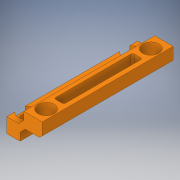
# Autodesk Inventor part: Block_3-8
Saved by Autodesk Inventor 2019 (Build 230136000, 136)
## iProperties
Created: 2019-03-07
Part Number: Block_3-8
Material: Aluminum 6061
Document SubType Name: Modeling
Designer: Delta
Density: 2.7 g/cm^3
Appearance: Orange
Mass: 102.344 g
Surface Area: 217.101 cm^2
Volume: 37.9051 cm^3
Author: Delta
Autodesk Inventor part; units mm, degrees
ref_plane "YZ Plane" through (0, 0, 0) normal (1, 0, 0) x (0, 1, 0)
ref_plane "XZ Plane" through (0, 0, 0) normal (0, 1, 0) x (-1, 0, 0)
ref_plane "XY Plane" through (0, 0, 0) normal (0, 0, 1) x (1, 0, 0)
sketch "Sketch1" plane through (0, 0, 0) normal (0, 0, 1) x (1, 0, 0)
  line L0 (0, 0) -> (0, 14.351)
  line L1 (0, 0) -> (14.351, 0) construction
  line L2 (0, 14.351) -> (16.51, 14.351)
  line L3 (16.51, 14.351) -> (16.51, 27.051)
  line L4 (16.51, 27.051) -> (34.29, 27.051)
  line L5 (34.29, 27.051) -> (34.29, 12.7)
  line L6 (34.29, 12.7) -> (12.7, 12.7)
  line L7 (12.7, 12.7) -> (12.7, 0)
  line L8 (0, 0) -> (12.7, 0)
  dimension "d0" = 14.351
  dimension "d2" = 16.51
  dimension "d6" = 17.78
  dimension "d9" = 21.59
  dimension "d47" = 14.351
  dimension "d49" = 12.7
  constraints: 18 end point, 6 perpendicular, 2 horizontal, 1 collinear, 1 point on line, 1 vertical
  measures "d0" distance of L0.start L0.end
  measures "d2" distance of L0.end L2.end
  measures "d6" distance of L3.end L4.end
  measures "d9" distance of L5.end L6.end
  measures "d47" distance of L4.end L5.end
  measures "d49" distance of L2.end L3.end
extrude "Extrusion1" add sketch "Sketch1" along normal blind 127
sketch "Sketch3" plane through (16.51, 27.051, 0) normal (0, 1, 0) x (1, 0, 0)
  line L0 (0, -127) -> (-16.51, -127) projected
  line L1 (-16.51, 0) -> (0, 0) projected
  line L2 (-16.51, 0) -> (-16.51, -127) projected
  point P0 (-10.16, -12.7)
  point P1 (-10.16, -114.3)
  dimension "d25" = 12.7
  dimension "d26" = 12.7
  dimension "d27" = 6.35
  dimension "d28" = 6.35
  measures "d25" distance from line of L0 point (-10.16, -114.3)
  measures "d26" distance from line of L1 point (-10.16, -12.7)
  measures "d27" distance from line of point (-10.16, -114.3) L2
  measures "d28" distance from line of point (-10.16, -12.7) L2
hole "Hole2" at (6.35, 27.051, 12.7) at (6.35, 27.051, 114.3) direction (0, -1, 0) diameter 9.525 end through all
sketch "Sketch4" plane through (16.51, 27.051, 0) normal (0, 1, 0) x (1, 0, 0)
  line L0 (17.78, 0) -> (17.78, -127) projected
  line L1 (17.78, -127) -> (0, -127) projected
  line L2 (0, 0) -> (17.78, 0) projected
  line L3 (0, 0) -> (0, -127) projected
  point P0 (-16.51, 0)
  point P1 (8.89, -12.7)
  point P2 (8.89, -114.3)
  dimension "d36" = 8.89
  dimension "d37" = 12.7
  dimension "d38" = 12.7
  dimension "d48" = 17.78
  constraints: 1 vertical alignment
  measures "d36" distance from line of L0 point (8.89, -12.7)
  measures "d37" distance from line of L1 point (8.89, -114.3)
  measures "d38" distance from line of L2 point (8.89, -12.7)
  measures "d48" distance between parallel lines of L0 L3
hole "Hole3" at (25.4, 27.051, 12.7) at (25.4, 27.051, 114.3) direction (0, -1, 0) diameter 15.875 end through all
sketch "Sketch5" plane through (16.51, 27.051, 0) normal (0, 1, 0) x (1, 0, 0)
  line L0 (3.81, -101.6) -> (13.335, -101.6)
  line L1 (13.335, -101.6) -> (13.335, -25.4)
  line L2 (13.335, -25.4) -> (3.81, -25.4)
  line L3 (3.81, -25.4) -> (3.81, -101.6)
  line L4 (17.78, -127) -> (0, -127) projected
  line L5 (17.78, 0) -> (17.78, -127) projected
  line L6 (0, 0) -> (17.78, 0) projected
  point P0 (-16.51, 0)
  dimension "d50" = 25.4
  dimension "d51" = 4.445
  dimension "d52" = 25.4
  dimension "d53" = 9.525
  constraints: 8 end point, 2 parallel, 1 horizontal, 1 perpendicular
  measures "d50" distance between parallel lines of L0 L4
  measures "d51" distance between parallel lines of L5 L1
  measures "d52" distance between parallel lines of L6 L2
  measures "d53" distance between parallel lines of L3 L1
extrude "Extrusion2" cut sketch "Sketch5" against normal blind 25.4
sketch "Sketch6" plane through (0, 0, 0) normal (0, -1, 0) x (1, 0, 0)
  line L0 (3.81, 25.4) -> (8.89, 25.4)
  line L1 (8.89, 25.4) -> (8.89, 101.6)
  line L2 (8.89, 101.6) -> (3.81, 101.6)
  line L3 (3.81, 101.6) -> (3.81, 25.4)
  line L4 (20.32, 101.6) -> (29.845, 101.6) projected
  line L5 (29.845, 25.4) -> (20.32, 25.4) projected
  line L6 (0, 0) -> (0, 127) projected
  line L7 (12.7, 0) -> (12.7, 127) projected
  dimension "d57" = 3.81
  dimension "d58" = 3.81
  constraints: 8 end point, 2 collinear, 2 parallel, 1 horizontal, 1 perpendicular
  measures "d57" distance between parallel lines of L6 L3
  measures "d58" distance between parallel lines of L7 L1
extrude "Extrusion3" cut sketch "Sketch6" against normal blind 25.4
fillet "Fillet1" radius 1.905 8 edges at (20.32, 19.8755, 25.4) (29.845, 19.8755, 25.4) (20.32, 19.8755, 101.6) (29.845, 19.8755, 101.6) (3.81, 7.1755, 101.6) (8.89, 7.1755, 101.6) (8.89, 7.1755, 25.4) (3.81, 7.1755, 25.4)
chamfer "Chamfer1" distance 5.08 angle 45 2 edges at (16.51, 14.351, 63.5) (12.7, 12.7, 63.5)
sketch "Sketch7" plane through (0, 14.351, 127) normal (0, 1, 0) x (1, 0, 0)
  circle A0 centre (6.35, 114.3) radius 4.7625 projected
  circle A1 centre (6.35, 114.3) radius 8.001
  circle A2 centre (6.35, 12.7) radius 4.7625 projected
  circle A3 centre (6.35, 12.7) radius 8.001
  point P0 (0, 127)
  dimension "d65" = 16.002
  dimension "d66" = 16.002
  constraints: 2 centre point, 2 coincident
  measures "d65" diameter of A1
  measures "d66" diameter of A3
extrude "Extrusion4" cut sketch "Sketch7" against normal blind 3.81
sketch "Sketch8" plane through (0, 14.351, 0) normal (0, 1, 0) x (1, 0, 0)
  arc A0 (0, -17.5676) -> (11.43, -18.8814) centre (6.35, -12.7) ccw projected
  circle A1 centre (6.35, -12.7) radius 8.001
  arc A2 (11.43, -108.1186) -> (0, -109.4324) centre (6.35, -114.3) ccw projected
  circle A3 centre (6.35, -114.3) radius 8.001
  point P0 (0, 0)
  constraints: 2 centre point, 2 coincident
extrude "Extrusion5" cut sketch "Sketch8" along normal blind 3.81
chamfer "Chamfer2" distance 2.54 angle 45 1 edges at (34.29, 12.7, 63.5)
equation "\"d0\" = d47"
equation "\"d26\" = d25"
equation "\"d28\" = d27"
equation "\"d36\" = 0.5 * d48"
equation "\"d38\" = d37"
equation "\"d58\" = d57"
body "Solid1"
